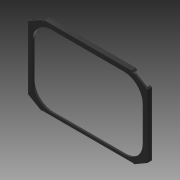
# Autodesk Inventor part: RubberLidSeal
Saved by Autodesk Inventor 2014 SP2 (Build 180246200, 246)
## iProperties
Created: 2015-09-16
Part Number: RubberLidSeal
Material: Rubber
Document SubType Name: Modeling
Designer: Lukasz Szmit
Density: 0.93 g/cm^3
Appearance: Rubber - Black - Version 1.1
Mass: 2.41449 g
Surface Area: 41.9671 cm^2
Volume: 2.59623 cm^3
Author: Lukasz Szmit
Autodesk Inventor part; units mm, degrees
ref_plane "YZ Plane" through (0, 0, 0) normal (1, 0, 0) x (0, 1, 0)
ref_plane "XZ Plane" through (0, 0, 0) normal (0, 1, 0) x (-1, 0, 0)
ref_plane "XY Plane" through (0, 0, 0) normal (0, 0, 1) x (1, 0, 0)
sketch "Seal Outline" plane through (0, 0, 0) normal (0, 1, 0) x (-1, 0, 0)
  line L0 (-48, 41.5) -> (48, 41.5)
  line L1 (62, 34.9661) -> (62, -34.9661)
  line L2 (-62, -34.9661) -> (-62, 34.9661)
  line L3 (62, 41.5045) -> (62, 41.5)
  arc A0 (-49.8748, 41.9666) -> (-48, 41.5) centre (-48, 45.5) ccw
  arc A1 (48, 41.5) -> (49.8748, 41.9666) centre (48, 45.5) ccw
  line L4 (48, 41.5) -> (37.7809, 41.4967)
  line L5 (-49.8748, 41.9666) -> (-62, 34.9661)
  line L6 (49.8748, 41.9666) -> (62, 34.9661)
  line L7 (62, -41.5045) -> (62, -41.5)
  arc A2 (49.8748, -41.9666) -> (48, -41.5) centre (48, -45.5) ccw
  line L8 (48, -41.5) -> (37.7809, -41.4967)
  line L9 (-48, -41.5) -> (48, -41.5)
  arc A3 (-48, -41.5) -> (-49.8748, -41.9666) centre (-48, -45.5) ccw
  line L10 (-49.8748, -41.9666) -> (-62, -34.9661)
  line L11 (49.8748, -41.9666) -> (62, -34.9661)
  line L12 (-39, 38.5) -> (39, 38.5)
  line L13 (59, 18.5) -> (59, -18.5)
  line L14 (39, -38.5) -> (-39, -38.5)
  line L15 (-59, -18.5) -> (-59, 18.5)
  arc A4 (-59, -18.5) -> (-39, -38.5) centre (-39, -18.5) ccw
  arc A5 (-39, 38.5) -> (-59, 18.5) centre (-39, 18.5) ccw
  arc A6 (59, 18.5) -> (39, 38.5) centre (39, 18.5) ccw
  arc A7 (39, -38.5) -> (59, -18.5) centre (39, -18.5) ccw
  point P0 (0, 0)
  dimension "d6" = 124
  dimension "d7" = 96
  dimension "d14" = 83
  dimension "d15" = 4
  dimension "d16" = 4
  dimension "d17" = 4
  dimension "d18" = 4
  dimension "d19" = 60
  dimension "d20" = 120
  dimension "d21" = 89.982
  dimension "d22" = 89.982
  dimension "d23" = 90
  dimension "d24" = 0
  dimension "d25" = 122.5631
  dimension "d26" = 122.5631
  dimension "d27" = 62
  dimension "d28" = 62
  dimension "d29" = 61.2816
  dimension "d30" = 61.2816
  dimension "d31" = 41.4847
  dimension "d32" = 41.4847
  dimension "d33" = 41.5
  dimension "d34" = 5.6585
  dimension "d35" = 66.2216
  dimension "d36" = 24.2191
  dimension "d37" = 24.2191
  dimension "d38" = 110
  dimension "d39" = 78
  dimension "d40" = 20
  dimension "d41" = 37
  dimension "d43" = 3
  dimension "d44" = 3
  constraints: 32 end point, 16 point on circle, 12 tangent, 8 centre point, 4 equal radius, 4 parallel, 3 perpendicular, 2 point on line, 1 vertical
  measures "d6" distance between parallel lines of L1 L2
  measures "d7" distance of L0.start L4.start
  measures "d14" distance between parallel lines of L9 L0
  measures "d15" radius of A0
  measures "d16" radius of A1
  measures "d17" radius of A3
  measures "d18" radius of A2
  measures "d19" angle of L3 L6
  measures "d20" angle of L3 L11
  measures "d21" angle of L3 L4
  measures "d22" angle of L8 L3
  measures "d23" angle of L3 L0
  measures "d24" distance between parallel lines of L7 L1
  measures "d25" distance between parallel lines of L6 L10
  measures "d26" distance between parallel lines of L11 L5
  measures "d27" distance from line of point (0, 0) L3
  measures "d28" distance from line of point (0, 0) L1
  measures "d29" distance from line of point (0, 0) L6
  measures "d30" distance from line of point (0, 0) L11
  measures "d31" distance from line of point (0, 0) L4
  measures "d32" distance from line of point (0, 0) L8
  measures "d33" distance from line of point (0, 0) L0
  measures "d34" distance from line of L3.end L6
  measures "d35" distance from line of L7.end L6
  measures "d36" distance from line of L4.end L1
  measures "d37" distance from line of L8.end L3
  measures "d38" distance from line of L9.start L3
  measures "d39" distance of A6.centre A5.centre
  measures "d40" radius of A6
  measures "d41" distance of A7.centre A6.centre
  measures "d43" distance between parallel lines of L2 L15
  measures "d44" distance between parallel lines of L9 L14
extrude "Extrusion1" add sketch "Seal Outline" along normal blind 1.85
sketch "Sketch2" plane through (0, 0, 0) normal (0, -1, 0) x (1, 0, 0)
  line L0 (62, 34.9661) -> (62, -34.9661) projected
  line L1 (-48, 41.5) -> (48, 41.5) projected
  line L2 (-62, -34.9661) -> (-62, 34.9661) projected
  line L3 (-48, 41.5) -> (-46.9319, 43.35)
  line L4 (-46.9319, 43.35) -> (46.9319, 43.35)
  line L5 (46.9319, 43.35) -> (48, 41.5)
  line L6 (-62, 34.9661) -> (-63.85, 33.898)
  line L7 (-63.85, 33.898) -> (-63.85, -33.898)
  line L8 (-63.85, -33.898) -> (-62, -34.9661)
  line L9 (62, 34.9661) -> (63.85, 33.898)
  line L10 (63.85, 33.898) -> (63.85, -33.898)
  line L11 (63.85, -33.898) -> (62, -34.9661)
  point P0 (-48, -41.5)
  point P1 (48, -41.5)
  dimension "d47" = 120
  dimension "d49" = 120
  dimension "d50" = 1.85
  dimension "d51" = 120
  dimension "d55" = 120
  dimension "d57" = 1.85
  dimension "d58" = 120
  dimension "d59" = 120
  dimension "d60" = 1.85
  constraints: 18 end point, 3 parallel
  measures "d47" angle of L1 L3
  measures "d49" angle of L1 L5
  measures "d50" distance between parallel lines of L1 L4
  measures "d51" angle of L2 L6
  measures "d55" angle of L2 L8
  measures "d57" distance between parallel lines of L7 L2
  measures "d58" angle of L0 L9
  measures "d59" angle of L0 L11
  measures "d60" distance between parallel lines of L0 L10
extrude "Extrusion3" add sketch "Sketch2" against normal blind 5
equation "\"d49\" = d47"
equation "\"d51\" = d47"
equation "\"d55\" = d47"
equation "\"d57\" = d50"
equation "\"d58\" = d47"
equation "\"d59\" = d47"
equation "\"d60\" = d50"
body "Solid1"
